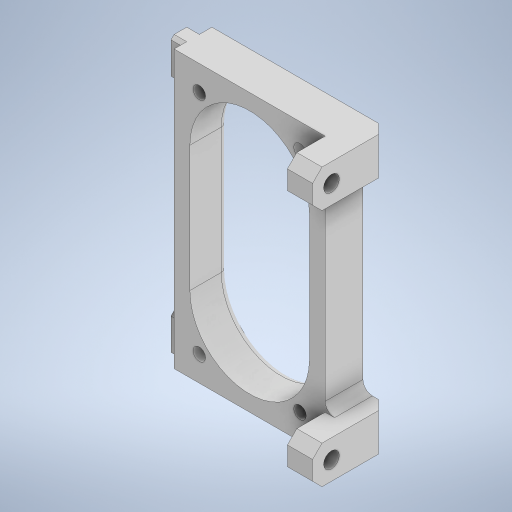
# Autodesk Inventor part: 스피커 조립부품
Saved by Autodesk Inventor 2023 (Build 270158000, 158)
## iProperties
Created: 2022-06-09
Part Number: 스피커 조립부품
Material: 일반
Document SubType Name: Modeling
Designer: fly01
Density: 1 g/cm^3
Appearance: 기본값
Author: fly01
Autodesk Inventor part; units mm, degrees
ref_plane "YZ Plane" through (0, 0, 0) normal (1, 0, 0) x (0, 1, 0)
ref_plane "XZ Plane" through (0, 0, 0) normal (0, 1, 0) x (-1, 0, 0)
ref_plane "XY Plane" through (0, 0, 0) normal (0, 0, 1) x (1, 0, 0)
sketch "스케치1" plane through (0, 0, 0) normal (0, 0, 1) x (1, 0, 0)
  line L0 (-12, 22) -> (12, 22)
  line L1 (12, 22) -> (12, -22)
  line L2 (12, -22) -> (-12, -22)
  line L3 (-12, -22) -> (-12, 22)
  line L4 (-12, 22) -> (12, -22) construction
  line L5 (12, 22) -> (-12, -22) construction
  line L6 (9.5, -10) -> (9.5, 10)
  line L7 (-9.5, 10) -> (-9.5, -10)
  line L8 (-9.5, -19.5) -> (9.5, 19.5) construction
  line L9 (9.5, -19.5) -> (-9.5, 19.5) construction
  arc A0 (0, 19.5) -> (-9.5, 10) centre (0, 10) ccw
  arc A1 (9.5, 10) -> (0, 19.5) centre (0, 10) ccw
  arc A2 (-9.5, -10) -> (0, -19.5) centre (0, -10) ccw
  arc A3 (0, -19.5) -> (9.5, -10) centre (0, -10) ccw
  point P0 (0, 0)
  point P1 (0, -19.5)
  point P2 (0, 19.5)
  dimension "d0" = 24
  dimension "d1" = 44
  dimension "d2" = 19
  dimension "d3" = 39
  dimension "d4" = 9.5
  dimension "d5" = 9.5
  constraints: 20 end point, 8 point on circle, 4 centre point, 4 point on line, 4 tangent, 3 midpoint, 3 parallel, 2 concentric, 1 horizontal, 1 perpendicular, 1 vertical, 14 other
  measures "d0" distance of L1.end L2.end
  measures "d1" distance of L0.end L1.end
  measures "d2" distance of L9.end L8.end
  measures "d3" distance of L8.end L9.start
  measures "d4" radius of A0
  measures "d5" radius of A2
extrude "돌출1" add sketch "스케치1" along normal blind 6
sketch "스케치2" plane through (0, 0, 0) normal (0, 0, -1) x (-1, 0, 0)
  line L0 (-8, -18) -> (8, -18)
  line L1 (8, -18) -> (8, 18)
  line L2 (8, 18) -> (-8, 18)
  line L3 (-8, 18) -> (-8, -18)
  line L4 (-8, -18) -> (8, 18) construction
  line L5 (8, -18) -> (-8, 18) construction
  circle A0 centre (-8, 18) radius 1
  circle A1 centre (8, 18) radius 1
  circle A2 centre (8, -18) radius 1
  circle A3 centre (-8, -18) radius 1
  point P0 (0, 0)
  dimension "d8" = 16
  dimension "d9" = 36
  dimension "d10" = 2
  dimension "d11" = 2
  dimension "d12" = 2
  dimension "d13" = 2
  constraints: 12 end point, 4 centre point, 4 coincident, 2 midpoint, 2 parallel, 1 horizontal, 1 perpendicular
  measures "d8" distance of L2.end L1.end
  measures "d9" distance of L0.end L1.end
  measures "d10" diameter of A0
  measures "d11" diameter of A1
  measures "d12" diameter of A2
  measures "d13" diameter of A3
extrude "돌출2" cut sketch "스케치2" against normal blind 6 contours L3 A3 L0 | L0 A3 L3 | A2 L1 L0 | L0 L1 A2 | A0 L2 L3 | L3 L2 A0 | A1 L2 L1 | L1 L2 A1
fillet "모깎기1" radius 1 4 edges at (9.5, 0, 0) (0, -19.5, 0) (-9.5, 0, 0) (0, 19.5, 0)
fillet "모깎기2" radius 0.3 12 edges at (7.2929, 17.2929, 0.0175) (8.7714, 18.6364, 0) (7.0046, 17.9045, 0) (-7.2929, 17.2929, 0.0175) (-7.9045, 18.9954, 0) (-8.6364, 17.2286, 0) (-7.2929, -17.2929, 0.0175) (-7.9045, -18.9954, 0) (-8.6364, -17.2286, 0) (7.2929, -17.2929, 0.0175) (7.0046, -17.9045, 0) (8.7714, -18.6364, 0)
sketch "스케치3" plane through (-12, -22, 0) normal (-1, 0, 0) x (0, 0, 1)
  line L0 (1.5, 0) -> (1.5, 44)
  line L1 (1.5, 44) -> (4.5, 44)
  line L2 (4.5, 44) -> (4.5, 38)
  line L3 (4.5, 38) -> (1.5, 38)
  line L4 (1.5, 38) -> (1.5, 44)
  line L5 (0, 22) -> (6, 22)
  line L6 (6, 12) -> (6, 32) projected
  line L7 (1.5, 0) -> (4.5, 0)
  line L8 (4.5, 0) -> (4.5, 6)
  line L9 (4.5, 6) -> (1.5, 6)
  line L10 (1.5, 6) -> (1.5, 0)
  line L11 (0, 44) -> (0, 0) projected
  point P0 (1.5, 6)
  dimension "d18" = 3
  dimension "d19" = 6
  dimension "d22" = 1.5
  constraints: 18 end point, 3 symmetric about line, 2 parallel, 1 horizontal, 1 midpoint, 1 perpendicular, 3 other
  measures "d18" distance of L2.end L3.end
  measures "d19" distance of L1.end L2.end
extrude "돌출3" add sketch "스케치3" along normal blind 2
chamfer "모따기1" distance 0.5 angle 45 8 edges at (-13, 22, 4.5) (-13, 16, 4.5) (-13, 16, 1.5) (-13, 22, 1.5) (-13, -16, 4.5) (-13, -16, 1.5) (-13, -22, 4.5) (-13, -22, 1.5)
sketch "스케치4" plane through (12, -22, 0) normal (1, 0, 0) x (0, 0, -1)
  line L0 (0, 44) -> (0, 0) projected
  line L1 (0, 44) -> (-12, 44)
  line L2 (-12, 44) -> (-12, 38)
  line L3 (-12, 38) -> (0, 38)
  line L4 (0, 38) -> (0, 44)
  line L5 (0, 0) -> (-12, 0)
  line L6 (-12, 0) -> (-12, 6)
  line L7 (-12, 6) -> (0, 6)
  line L8 (0, 6) -> (0, 0)
  point P0 (0, 22)
  point P1 (0, 6)
  point P2 (0, 38)
  dimension "d26" = 6
  dimension "d27" = 12
  dimension "d28" = 12
  dimension "d29" = 6
  constraints: 16 end point, 4 parallel, 2 horizontal, 2 perpendicular
  measures "d26" distance of L1.end L2.end
  measures "d27" distance of L2.end L3.end
  measures "d28" distance of L6.end L7.end
  measures "d29" distance of L5.end L6.end
extrude "돌출4" add sketch "스케치4" along normal blind 4
fillet "모깎기3" radius 1.5 2 edges at (12, 16, 3) (12, -16, 3)
sketch "스케치5" plane through (16, -22, 0) normal (1, 0, 0) x (0, 0, -1)
  line L0 (-12, 38) -> (-6, 38) projected
  line L1 (-12, 44) -> (-12, 38) projected
  line L2 (-6, 38) -> (-12, 44) construction
  line L3 (-6, 6) -> (-6, 7.5) projected
  line L4 (-6, 6) -> (0, 6) projected
  line L5 (0, 6) -> (0, 7.5) projected
  line L6 (0, 7.5) -> (-6, 7.5) projected
  line L7 (-6, 6) -> (-12, -0.0965) construction
  circle A0 centre (-9, 2.9517) radius 1.25
  circle A1 centre (-9, 41) radius 1.25
  point P0 (0, 22)
  dimension "d33" = 2.5
  dimension "d34" = 2.5
  constraints: 4 end point, 2 centre point, 2 midpoint
  measures "d33" diameter of A0
  measures "d34" diameter of A1
extrude "돌출5" cut sketch "스케치5" against normal blind 4 contours A0 | A1
chamfer "모따기2" distance 1.5 angle 45 4 edges at (14, 22, 12) (14, 16, 12) (14, -16, 12) (14, -22, 12)
chamfer "모따기3" distance 1.5 angle 45 2 edges at (16, -19, 0) (16, 19, 0)
